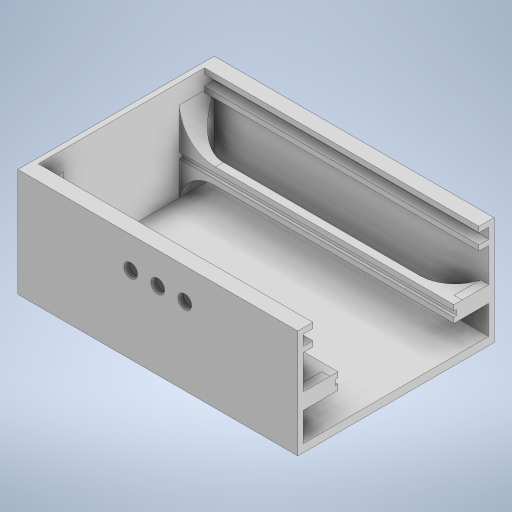
# Autodesk Inventor part: Remote
Saved by Autodesk Inventor 2023 (Build 270158000, 158)
## iProperties
Created: 2023-03-27
Part Number: Remote
Material: Générique
Document SubType Name: Modeling
Designer: eleves
Density: 1 g/cm^3
Appearance: Par défaut
Author: eleves
Autodesk Inventor part; units mm, degrees
ref_plane "YZ Plane" through (0, 0, 0) normal (1, 0, 0) x (0, 1, 0)
ref_plane "XZ Plane" through (0, 0, 0) normal (0, 1, 0) x (-1, 0, 0)
ref_plane "XY Plane" through (0, 0, 0) normal (0, 0, 1) x (1, 0, 0)
sketch "Esquisse1" plane through (0, 0, 0) normal (0, 1, 0) x (-1, 0, 0)
  line L0 (-49.75, -34.3) -> (49.75, -34.3)
  line L1 (49.75, -34.3) -> (49.75, 34.3)
  line L2 (49.75, 34.3) -> (-49.75, 34.3)
  line L3 (-49.75, 34.3) -> (-49.75, -34.3)
  line L4 (-49.75, -34.3) -> (49.75, 34.3) construction
  line L5 (49.75, -34.3) -> (-49.75, 34.3) construction
  line L6 (-51.75, 36.3) -> (51.75, 36.3)
  line L7 (51.75, 36.3) -> (51.75, -36.3)
  line L8 (51.75, -36.3) -> (-51.75, -36.3)
  line L9 (-51.75, -36.3) -> (-51.75, 36.3)
  point P0 (0, 0)
  dimension "d0" = 99.5
  dimension "d1" = 68.6
  dimension "d2" = 2
  constraints: 20 end point, 4 parallel, 2 midpoint, 2 perpendicular, 1 horizontal, 3 other
  measures "d0" distance of L1.end L2.end
  measures "d1" distance of L0.end L1.end
  measures "d2" distance between parallel lines of L2 L6
extrude "Extrusion1" add sketch "Esquisse1" along normal blind 3 contours L3 L2 L1 L0
extrude "Extrusion2" add sketch "Esquisse1" along normal blind 40
sketch "Esquisse2" plane through (51.75, 0, 36.3) normal (1, 0, 0) x (0, 0, -1)
  line L0 (2, 40) -> (70.6, 40)
  line L1 (70.6, 40) -> (70.6, 3)
  line L2 (70.6, 3) -> (2, 3)
  line L3 (2, 3) -> (2, 40)
  line L4 (2, 3) -> (70.6, 3) projected
  point P0 (36.3, 0)
  constraints: 8 end point, 2 parallel, 1 collinear, 1 horizontal, 1 perpendicular
extrude "Extrusion3" cut sketch "Esquisse2" against normal blind 40
sketch "Esquisse3" plane through (51.75, 0, 36.3) normal (1, 0, 0) x (0, 0, -1)
  line L0 (2, 3) -> (2, 40) projected
  line L1 (2, 40) -> (5.5781, 40)
  line L2 (5.5781, 40) -> (5.5781, 38)
  line L3 (5.5781, 38) -> (2, 38)
  line L4 (2, 38) -> (2, 40)
  line L5 (2, 34.1) -> (5.5781, 34.1)
  line L6 (5.5781, 34.1) -> (5.5781, 32.1)
  line L7 (5.5781, 32.1) -> (2, 32.1)
  line L8 (2, 32.1) -> (2, 34.1)
  line L9 (36.3, 0) -> (36.3, 40) construction
  line L10 (2, 40) -> (70.6, 40) construction
  line L11 (70.6, 3) -> (70.6, 40)
  line L12 (70.6, 40) -> (67.0219, 40)
  line L13 (67.0219, 40) -> (67.0219, 38)
  line L14 (67.0219, 38) -> (70.6, 38)
  line L15 (70.6, 38) -> (70.6, 40)
  line L16 (70.6, 34.1) -> (67.0219, 34.1)
  line L17 (67.0219, 34.1) -> (67.0219, 32.1)
  line L18 (67.0219, 32.1) -> (70.6, 32.1)
  line L19 (70.6, 32.1) -> (70.6, 34.1)
  line L20 (70.6, 40) -> (2, 40) construction
  point P0 (2, 32.1)
  point P1 (2, 38)
  dimension "d9" = 2
  dimension "d10" = 2
  dimension "d11" = 3.9
  constraints: 38 end point, 10 symmetric about line, 4 parallel, 2 horizontal, 2 perpendicular, 2 point on line, 1 midpoint
  measures "d9" distance of L1.end L2.end
  measures "d10" distance of L5.end L6.end
  measures "d11" distance between parallel lines of L5 L3
extrude "Extrusion4" add sketch "Esquisse3" against normal up to surface (101.5 mm away)
sketch "Esquisse4" plane through (-49.75, 3, 34.3) normal (1, 0, 0) x (0, 0, -1)
  line L0 (56.75, 12.5643) -> (11.85, 12.5643) construction
  line L1 (11.85, 12.5643) -> (11.85, 14.5643) construction
  line L2 (11.85, 14.5643) -> (56.75, 14.5643) construction
  line L3 (56.75, 14.5643) -> (56.75, 12.5643) construction
  line L4 (56.75, 12.5643) -> (11.85, 14.5643) construction
  line L5 (11.85, 12.5643) -> (56.75, 14.5643) construction
  line L6 (12.85, 12.5643) -> (12.85, 10.5643)
  line L7 (12.85, 10.5643) -> (9.85, 10.5643)
  line L8 (9.85, 10.5643) -> (9.85, 16.5643)
  line L9 (9.85, 16.5643) -> (12.85, 16.5643)
  line L10 (12.85, 14.5643) -> (12.85, 16.5643)
  line L11 (12.85, 12.5643) -> (11.85, 12.5643)
  line L12 (11.85, 14.5643) -> (11.85, 12.5643)
  line L13 (11.85, 14.5643) -> (12.85, 14.5643)
  line L14 (34.3, 13.5643) -> (34.3, 18.2352) construction
  line L15 (56.75, 12.5643) -> (56.75, 14.5643) construction
  line L16 (55.75, 12.5643) -> (55.75, 10.5643)
  line L17 (55.75, 10.5643) -> (58.75, 10.5643)
  line L18 (58.75, 10.5643) -> (58.75, 16.5643)
  line L19 (58.75, 16.5643) -> (55.75, 16.5643)
  line L20 (55.75, 14.5643) -> (55.75, 16.5643)
  line L21 (55.75, 12.5643) -> (56.75, 12.5643)
  line L22 (56.75, 14.5643) -> (56.75, 12.5643)
  line L23 (56.75, 14.5643) -> (55.75, 14.5643)
  point P0 (34.3, -3)
  dimension "d14" = 44.9
  dimension "d15" = 2
  dimension "d16" = 2
  dimension "d17" = 1
  dimension "d18" = 2
  dimension "d19" = 2
  constraints: 48 end point, 6 perpendicular, 6 symmetric about line, 2 collinear, 2 horizontal, 2 midpoint, 2 parallel, 2 point on line, 2 vertical
  measures "d14" distance of L0.start L0.end
  measures "d15" distance of L0.end L1.end
  measures "d16" distance between parallel lines of L8 L1
  measures "d17" distance between parallel lines of L10 L1
  measures "d18" distance between parallel lines of L9 L2
  measures "d19" distance between parallel lines of L0 L7
extrude "Extrusion5" add sketch "Esquisse4" along normal up to surface (101.5 mm away)
fillet "Congé1" radius 13.25 6 edges at (-49.75, 19.5643, 22.95) (-49.75, 19.5643, -22.95) (-49.75, 13.5643, -22.95) (-49.75, 13.5643, 22.95) (-49.75, 16.5643, -24.45) (-49.75, 16.5643, 24.45)
sketch "Esquisse5" plane through (51.75, 0, 36.3) normal (1, 0, 0) x (0, 0, -1)
  line L0 (11.85, 13.5633) -> (11.85, 19.5718) projected
  line L1 (2, 3) -> (2, 32.1) projected
  line L2 (11.85, 19.5718) -> (2, 19.5718)
  line L3 (2, 19.5718) -> (2, 13.5643)
  line L4 (2, 13.5643) -> (11.85, 13.5643)
  line L5 (11.85, 13.5643) -> (11.85, 19.5718)
  line L6 (14.85, 13.5643) -> (11.85, 13.5643) projected
  line L7 (36.3, 0) -> (36.3, 40) construction
  line L8 (72.6, 40) -> (0, 40) construction
  line L9 (60.75, 13.5633) -> (60.75, 19.5718)
  line L10 (60.75, 19.5718) -> (70.6, 19.5718)
  line L11 (70.6, 19.5718) -> (70.6, 13.5643)
  line L12 (70.6, 13.5643) -> (60.75, 13.5643)
  line L13 (60.75, 13.5643) -> (60.75, 19.5718)
  line L14 (57.75, 13.5643) -> (60.75, 13.5643)
  point P0 (11.85, 13.5643)
  point P1 (2, 19.5718)
  constraints: 22 end point, 7 symmetric about line, 2 parallel, 1 collinear, 1 horizontal, 1 midpoint, 1 perpendicular, 1 point on line
extrude "Extrusion6" add sketch "Esquisse5" against normal blind 3
fillet "Congé2" radius 13.25 2 edges at (48.75, 16.5643, 24.45) (48.75, 16.5643, -24.45)
sketch "Esquisse6" plane through (-51.75, 0, 36.3) normal (0, 0, 1) x (1, 0, 0)
  line L0 (51.75, 0) -> (51.75, 40)
  line L1 (103.5, 40) -> (0, 40) projected
  circle A0 centre (51.75, 28.5321) radius 2.5
  circle A1 centre (61.75, 28.5321) radius 2.5
  circle A2 centre (41.75, 28.5321) radius 2.5
  dimension "d26" = 5
  dimension "d27" = 5
  dimension "d28" = 5
  dimension "d29" = 10
  dimension "d30" = 10
  constraints: 3 centre point, 2 end point, 1 midpoint, 1 point on line
  measures "d26" diameter of A0
  measures "d27" diameter of A2
  measures "d28" diameter of A1
  measures "d29" distance of A1.centre A0.centre
  measures "d30" distance of A2.centre A0.centre
extrude "Extrusion7" cut sketch "Esquisse6" against normal blind 3
